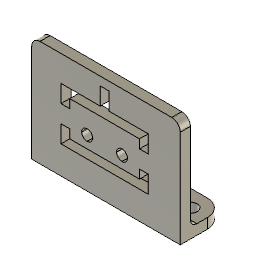
BrandalPilaR v6 (Autodesk Fusion 360 design; units mm, degrees)
Autodesk Fusion 360 part; units mm, degrees
sketch "Sketch1" plane through (0, 0, 0) normal (0, 0, 1) x (1, 0, 0)
  circle A0 centre (0, 0) radius 1.6
  circle A1 centre (0, 0) radius 4
  line L0 (0, 4) -> (20, 4)
  circle A2 centre (20, 0) radius 4
  line L1 (0, -4) -> (20, -4)
  circle A3 centre (20, 0) radius 1.6
  line L2 (-4, 0) -> (-4, -4)
  line L3 (-4, -4) -> (0, -4)
  line L4 (20, -4) -> (24, -4)
  line L5 (24, -4) -> (24, 0)
  dimension "d1" = 3.2
  dimension "d2" = 8
  dimension "d3" = 20
  constraint coincident A0.centre A1.centre
  constraint concentric A0 A1
  constraint coincident A1 L0.start
  constraint horizontal L0
  constraint coincident L0.end A2
  constraint tangent L0 A2
  constraint coincident A1 L1.start
  constraint coincident A2 L1.end
  constraint tangent A2 L1
  constraint horizontal L1
  constraint tangent A1 L1
  constraint tangent A1 L0
  constraint concentric A2 A3
  constraint equal A0 A3
  constraint coincident A1 L2.start
  constraint vertical L2
  constraint horizontal L3
  constraint tangent A1 L2
  constraint tangent A2 L4
  constraint coincident A2 L5.end
  constraint tangent A2 L5
  constraint vertical L5
  measures "d1" diameter of A0
  measures "d2" diameter of A1
  measures "d3" distance of L0.start L0.end
extrude "Extrude1" add sketch "Sketch1" along normal blind 2.4 contours A1 | A1 L0 A2 L1 | A1 L2 L3 | A2 | A2 L4 L5 picked at (-0.2296, -3.1849) picked at (12.0075, 0) picked at (-3.2141, -3.2141) picked at (18.4037, 2.7648) picked at (23.2141, -3.2141)
sketch "Sketch2" plane through (0, -4, 0) normal (0, -1, 0) x (1, 0, 0)
  line L0 (-4, 0) -> (24, 0)
  line L1 (24, 0) -> (24, 2.4)
  line L2 (24, 2.4) -> (-4, 2.4)
  line L3 (-4, 2.4) -> (-4, 0)
  line L4 (-11, 25) -> (24, 25)
  line L5 (24, 25) -> (24, 0)
  line L6 (-4, 0) -> (-11, 0)
  line L7 (-11, 0) -> (-11, 25)
  dimension "d11" = 25
  dimension "d12" = 35
  constraint coincident L0.end L1.start
  constraint perpendicular L0 L5
  constraint coincident L0.start L3.end
  constraint perpendicular L6 L7
  constraint horizontal L4
  constraint vertical L7
  measures "d11" distance of L6.end L4.start
  measures "d12" distance of L4.end L4.start
extrude "Extrude2" add sketch "Sketch2" along normal blind 2.4 contours L0 L1 L2 L3 L5 | L2 L3 L4 L5 L6 L7 picked at (14.6667, 0.8) picked at (3, 17.4667)
fillet "Fillet1" radius 2 2 edges at (24, -5.2, 25) (-11, -5.2, 25)
fillet "Fillet2" radius 1.5 1 edges at (10, -4, 2.4)
sketch "Sketch3" plane through (0, -6.4, 0) normal (0, -1, 0) x (1, 0, 0)
  arc A0 (-9, 25) -> (-11, 23) centre (-9, 23) ccw
  line L0 (-11, 23) -> (-11, 0)
  line L1 (-11, 0) -> (24, 0)
  line L2 (24, 0) -> (24, 23)
  arc A1 (24, 23) -> (22, 25) centre (22, 23) ccw
  line L3 (22, 25) -> (-9, 25)
  spline S0 degree 3 poles (-4.878, 0.7667) (-5.1447, 0.7667) (-5.3826, 0.824) (-5.5918, 0.9388) knots 0 0 0 0 1 1 1 1
  spline S1 degree 3 poles (-5.5918, 0.9388) (-5.801, 1.0535) (-5.9664, 1.2071) (-6.0879, 1.3994) knots 0 0 0 0 1 1 1 1
  spline S2 degree 3 poles (-6.0879, 1.3994) (-6.2094, 1.5952) (-6.2701, 1.8145) (-6.2701, 2.0575) knots 0 0 0 0 1 1 1 1
  spline S3 degree 3 poles (-6.2701, 2.0575) (-6.2701, 2.3005) (-6.2094, 2.5182) (-6.0879, 2.7105) knots 0 0 0 0 1 1 1 1
  spline S4 degree 3 poles (-6.0879, 2.7105) (-5.9664, 2.9062) (-5.801, 3.0615) (-5.5918, 3.1762) knots 0 0 0 0 1 1 1 1
  spline S5 degree 3 poles (-5.5918, 3.1762) (-5.3826, 3.291) (-5.1447, 3.3483) (-4.878, 3.3483) knots 0 0 0 0 1 1 1 1
  line L4 (-4.878, 3.3483) -> (-4.5642, 3.3483)
  line L5 (-4.5642, 3.3483) -> (-4.5642, 2.8523)
  line L6 (-4.5642, 2.8523) -> (-4.8882, 2.8523)
  spline S6 degree 3 poles (-4.8882, 2.8523) (-5.0434, 2.8523) (-5.1818, 2.8168) (-5.3033, 2.746) knots 0 0 0 0 1 1 1 1
  spline S7 degree 3 poles (-5.3033, 2.746) (-5.4214, 2.6784) (-5.5142, 2.584) (-5.5817, 2.4625) knots 0 0 0 0 1 1 1 1
  spline S8 degree 3 poles (-5.5817, 2.4625) (-5.6492, 2.341) (-5.6829, 2.206) (-5.6829, 2.0575) knots 0 0 0 0 1 1 1 1
  spline S9 degree 3 poles (-5.6829, 2.0575) (-5.6829, 1.909) (-5.6492, 1.774) (-5.5817, 1.6526) knots 0 0 0 0 1 1 1 1
  spline S10 degree 3 poles (-5.5817, 1.6526) (-5.5142, 1.5311) (-5.4214, 1.4349) (-5.3033, 1.364) knots 0 0 0 0 1 1 1 1
  spline S11 degree 3 poles (-5.3033, 1.364) (-5.1818, 1.2965) (-5.0434, 1.2628) (-4.8882, 1.2628) knots 0 0 0 0 1 1 1 1
  line L7 (-4.8882, 1.2628) -> (-4.5642, 1.2628)
  line L8 (-4.5642, 1.2628) -> (-4.5642, 0.7667)
  line L9 (-4.5642, 0.7667) -> (-4.878, 0.7667)
  line L10 (-4.057, 0.7667) -> (-4.057, 4.462)
  line L11 (-4.057, 4.462) -> (-3.4748, 4.462)
  line L12 (-3.4748, 4.462) -> (-3.4748, 3.0902)
  spline S12 degree 3 poles (-3.4748, 3.0902) (-3.3702, 3.2015) (-3.2487, 3.2825) (-3.1104, 3.3332) knots 0 0 0 0 1 1 1 1
  spline S13 degree 3 poles (-3.1104, 3.3332) (-2.972, 3.3838) (-2.8319, 3.4091) (-2.6902, 3.4091) knots 0 0 0 0 1 1 1 1
  spline S14 degree 3 poles (-2.6902, 3.4091) (-2.454, 3.4091) (-2.2532, 3.3585) (-2.0878, 3.2572) knots 0 0 0 0 1 1 1 1
  spline S15 degree 3 poles (-2.0878, 3.2572) (-1.9191, 3.1593) (-1.7909, 3.0227) (-1.7031, 2.8472) knots 0 0 0 0 1 1 1 1
  spline S16 degree 3 poles (-1.7031, 2.8472) (-1.6154, 2.6751) (-1.5715, 2.4777) (-1.5715, 2.2549) knots 0 0 0 0 1 1 1 1
  line L13 (-1.5715, 2.2549) -> (-1.5715, 0.7667)
  line L14 (-1.5715, 0.7667) -> (-2.1486, 0.7667)
  line L15 (-2.1486, 0.7667) -> (-2.1486, 2.2499)
  spline S17 degree 3 poles (-2.1486, 2.2499) (-2.1486, 2.3815) (-2.1806, 2.4962) (-2.2447, 2.5941) knots 0 0 0 0 1 1 1 1
  spline S18 degree 3 poles (-2.2447, 2.5941) (-2.3055, 2.6953) (-2.3865, 2.7729) (-2.4877, 2.8269) knots 0 0 0 0 1 1 1 1
  spline S19 degree 3 poles (-2.4877, 2.8269) (-2.5856, 2.8843) (-2.6953, 2.913) (-2.8168, 2.913) knots 0 0 0 0 1 1 1 1
  spline S20 degree 3 poles (-2.8168, 2.913) (-2.9315, 2.913) (-3.0395, 2.886) (-3.1407, 2.832) knots 0 0 0 0 1 1 1 1
  spline S21 degree 3 poles (-3.1407, 2.832) (-3.242, 2.778) (-3.323, 2.7021) (-3.3837, 2.6042) knots 0 0 0 0 1 1 1 1
  spline S22 degree 3 poles (-3.3837, 2.6042) (-3.4445, 2.5063) (-3.4748, 2.395) (-3.4748, 2.2701) knots 0 0 0 0 1 1 1 1
  line L16 (-3.4748, 2.2701) -> (-3.4748, 0.7667)
  line L17 (-3.4748, 0.7667) -> (-4.057, 0.7667)
  spline S23 degree 3 poles (0.1744, 0.7059) (-0.0719, 0.7059) (-0.2845, 0.7667) (-0.4634, 0.8882) knots 0 0 0 0 1 1 1 1
  spline S24 degree 3 poles (-0.4634, 0.8882) (-0.6423, 1.0097) (-0.7806, 1.1717) (-0.8785, 1.3741) knots 0 0 0 0 1 1 1 1
  spline S25 degree 3 poles (-0.8785, 1.3741) (-0.9729, 1.58) (-1.0202, 1.8061) (-1.0202, 2.0525) knots 0 0 0 0 1 1 1 1
  spline S26 degree 3 poles (-1.0202, 2.0525) (-1.0202, 2.3089) (-0.9662, 2.5384) (-0.8582, 2.7409) knots 0 0 0 0 1 1 1 1
  spline S27 degree 3 poles (-0.8582, 2.7409) (-0.7469, 2.9467) (-0.5899, 3.1087) (-0.3874, 3.2269) knots 0 0 0 0 1 1 1 1
  spline S28 degree 3 poles (-0.3874, 3.2269) (-0.1816, 3.3483) (0.0631, 3.4091) (0.3466, 3.4091) knots 0 0 0 0 1 1 1 1
  spline S29 degree 3 poles (0.3466, 3.4091) (0.6267, 3.4091) (0.8646, 3.3483) (1.0603, 3.2269) knots 0 0 0 0 1 1 1 1
  spline S30 degree 3 poles (1.0603, 3.2269) (1.2594, 3.1087) (1.4113, 2.9467) (1.5159, 2.7409) knots 0 0 0 0 1 1 1 1
  spline S31 degree 3 poles (1.5159, 2.7409) (1.6239, 2.5384) (1.6779, 2.3123) (1.6779, 2.0626) knots 0 0 0 0 1 1 1 1
  line L18 (1.6779, 2.0626) -> (1.6779, 0.7667)
  line L19 (1.6779, 0.7667) -> (1.0957, 0.7667)
  line L20 (1.0957, 0.7667) -> (1.0957, 1.2476)
  line L21 (1.0957, 1.2476) -> (1.0856, 1.2476)
  spline S32 degree 3 poles (1.0856, 1.2476) (1.035, 1.1531) (0.9692, 1.0637) (0.8882, 0.9793) knots 0 0 0 0 1 1 1 1
  spline S33 degree 3 poles (0.8882, 0.9793) (0.8072, 0.8983) (0.7077, 0.8325) (0.5895, 0.7819) knots 0 0 0 0 1 1 1 1
  spline S34 degree 3 poles (0.5895, 0.7819) (0.4714, 0.7313) (0.3331, 0.7059) (0.1744, 0.7059) knots 0 0 0 0 1 1 1 1
  spline S35 degree 3 poles (0.3314, 1.202) (0.4832, 1.202) (0.6148, 1.2391) (0.7262, 1.3134) knots 0 0 0 0 1 1 1 1
  spline S36 degree 3 poles (0.7262, 1.3134) (0.8409, 1.391) (0.9287, 1.4939) (0.9894, 1.6222) knots 0 0 0 0 1 1 1 1
  spline S37 degree 3 poles (0.9894, 1.6222) (1.0535, 1.7538) (1.0856, 1.9006) (1.0856, 2.0626) knots 0 0 0 0 1 1 1 1
  spline S38 degree 3 poles (1.0856, 2.0626) (1.0856, 2.2246) (1.0552, 2.368) (0.9945, 2.4929) knots 0 0 0 0 1 1 1 1
  spline S39 degree 3 poles (0.9945, 2.4929) (0.9338, 2.6211) (0.8477, 2.7223) (0.7363, 2.7966) knots 0 0 0 0 1 1 1 1
  spline S40 degree 3 poles (0.7363, 2.7966) (0.625, 2.8742) (0.4917, 2.913) (0.3364, 2.913) knots 0 0 0 0 1 1 1 1
  spline S41 degree 3 poles (0.3364, 2.913) (0.1744, 2.913) (0.0361, 2.8742) (-0.0787, 2.7966) knots 0 0 0 0 1 1 1 1
  spline S42 degree 3 poles (-0.0787, 2.7966) (-0.1934, 2.7223) (-0.2811, 2.6211) (-0.3419, 2.4929) knots 0 0 0 0 1 1 1 1
  spline S43 degree 3 poles (-0.3419, 2.4929) (-0.4026, 2.3646) (-0.433, 2.2195) (-0.433, 2.0575) knots 0 0 0 0 1 1 1 1
  spline S44 degree 3 poles (-0.433, 2.0575) (-0.433, 1.8989) (-0.4026, 1.7538) (-0.3419, 1.6222) knots 0 0 0 0 1 1 1 1
  spline S45 degree 3 poles (-0.3419, 1.6222) (-0.2811, 1.4939) (-0.1951, 1.391) (-0.0837, 1.3134) knots 0 0 0 0 1 1 1 1
  spline S46 degree 3 poles (-0.0837, 1.3134) (0.031, 1.2391) (0.1694, 1.202) (0.3314, 1.202) knots 0 0 0 0 1 1 1 1
  line L22 (2.3947, 0.7667) -> (2.3947, 4.3101)
  line L23 (2.3947, 4.3101) -> (4.3486, 4.3101)
  spline S47 degree 3 poles (4.3486, 4.3101) (4.5241, 4.3101) (4.6794, 4.2713) (4.8143, 4.1937) knots 0 0 0 0 1 1 1 1
  spline S48 degree 3 poles (4.8143, 4.1937) (4.9527, 4.1161) (5.0607, 4.0098) (5.1383, 3.8748) knots 0 0 0 0 1 1 1 1
  spline S49 degree 3 poles (5.1383, 3.8748) (5.2193, 3.7398) (5.2598, 3.5829) (5.2598, 3.404) knots 0 0 0 0 1 1 1 1
  spline S50 degree 3 poles (5.2598, 3.404) (5.2598, 3.2859) (5.2345, 3.1728) (5.1839, 3.0649) knots 0 0 0 0 1 1 1 1
  spline S51 degree 3 poles (5.1839, 3.0649) (5.1366, 2.9569) (5.0708, 2.8624) (4.9864, 2.7814) knots 0 0 0 0 1 1 1 1
  spline S52 degree 3 poles (4.9864, 2.7814) (4.9021, 2.7038) (4.8042, 2.643) (4.6928, 2.5992) knots 0 0 0 0 1 1 1 1
  spline S53 degree 3 poles (4.6928, 2.5992) (4.8211, 2.562) (4.9341, 2.4996) (5.032, 2.4119) knots 0 0 0 0 1 1 1 1
  spline S54 degree 3 poles (5.032, 2.4119) (5.1332, 2.3241) (5.2125, 2.2195) (5.2699, 2.098) knots 0 0 0 0 1 1 1 1
  spline S55 degree 3 poles (5.2699, 2.098) (5.3273, 1.9765) (5.356, 1.8466) (5.356, 1.7082) knots 0 0 0 0 1 1 1 1
  spline S56 degree 3 poles (5.356, 1.7082) (5.356, 1.526) (5.3138, 1.364) (5.2294, 1.2223) knots 0 0 0 0 1 1 1 1
  spline S57 degree 3 poles (5.2294, 1.2223) (5.1484, 1.0805) (5.0354, 0.9692) (4.8903, 0.8882) knots 0 0 0 0 1 1 1 1
  spline S58 degree 3 poles (4.8903, 0.8882) (4.7485, 0.8072) (4.5848, 0.7667) (4.3992, 0.7667) knots 0 0 0 0 1 1 1 1
  line L24 (4.3992, 0.7667) -> (2.3947, 0.7667)
  line L25 (2.9971, 1.3033) -> (4.2373, 1.3033)
  spline S59 degree 3 poles (4.2373, 1.3033) (4.3385, 1.3033) (4.4279, 1.3252) (4.5055, 1.3691) knots 0 0 0 0 1 1 1 1
  spline S60 degree 3 poles (4.5055, 1.3691) (4.5832, 1.4163) (4.6422, 1.4787) (4.6827, 1.5564) knots 0 0 0 0 1 1 1 1
  spline S61 degree 3 poles (4.6827, 1.5564) (4.7266, 1.6374) (4.7485, 1.7217) (4.7485, 1.8095) knots 0 0 0 0 1 1 1 1
  spline S62 degree 3 poles (4.7485, 1.8095) (4.7485, 1.9006) (4.7266, 1.9832) (4.6827, 2.0575) knots 0 0 0 0 1 1 1 1
  spline S63 degree 3 poles (4.6827, 2.0575) (4.6389, 2.1351) (4.5781, 2.1976) (4.5005, 2.2448) knots 0 0 0 0 1 1 1 1
  spline S64 degree 3 poles (4.5005, 2.2448) (4.4229, 2.292) (4.3317, 2.3157) (4.2271, 2.3157) knots 0 0 0 0 1 1 1 1
  line L26 (4.2271, 2.3157) -> (2.9971, 2.3157)
  line L27 (2.9971, 2.3157) -> (2.9971, 1.3033)
  line L28 (2.9971, 2.8269) -> (4.1613, 2.8269)
  spline S65 degree 3 poles (4.1613, 2.8269) (4.2558, 2.8269) (4.3402, 2.8489) (4.4144, 2.8928) knots 0 0 0 0 1 1 1 1
  spline S66 degree 3 poles (4.4144, 2.8928) (4.4921, 2.9366) (4.5511, 2.994) (4.5916, 3.0649) knots 0 0 0 0 1 1 1 1
  spline S67 degree 3 poles (4.5916, 3.0649) (4.6355, 3.1391) (4.6574, 3.2184) (4.6574, 3.3028) knots 0 0 0 0 1 1 1 1
  spline S68 degree 3 poles (4.6574, 3.3028) (4.6574, 3.3905) (4.6372, 3.4698) (4.5967, 3.5407) knots 0 0 0 0 1 1 1 1
  spline S69 degree 3 poles (4.5967, 3.5407) (4.5562, 3.6116) (4.4988, 3.6689) (4.4246, 3.7128) knots 0 0 0 0 1 1 1 1
  spline S70 degree 3 poles (4.4246, 3.7128) (4.3537, 3.7567) (4.271, 3.7786) (4.1765, 3.7786) knots 0 0 0 0 1 1 1 1
  line L29 (4.1765, 3.7786) -> (2.9971, 3.7786)
  line L30 (2.9971, 3.7786) -> (2.9971, 2.8269)
  spline S71 degree 3 poles (7.144, 0.7059) (6.8774, 0.7059) (6.6411, 0.765) (6.4353, 0.8831) knots 0 0 0 0 1 1 1 1
  spline S72 degree 3 poles (6.4353, 0.8831) (6.2295, 1.0046) (6.0658, 1.1666) (5.9443, 1.3691) knots 0 0 0 0 1 1 1 1
  spline S73 degree 3 poles (5.9443, 1.3691) (5.8262, 1.5749) (5.7671, 1.8044) (5.7671, 2.0575) knots 0 0 0 0 1 1 1 1
  spline S74 degree 3 poles (5.7671, 2.0575) (5.7671, 2.3106) (5.8262, 2.5384) (5.9443, 2.7409) knots 0 0 0 0 1 1 1 1
  spline S75 degree 3 poles (5.9443, 2.7409) (6.0658, 2.9467) (6.2295, 3.1087) (6.4353, 3.2269) knots 0 0 0 0 1 1 1 1
  spline S76 degree 3 poles (6.4353, 3.2269) (6.6411, 3.3483) (6.8774, 3.4091) (7.144, 3.4091) knots 0 0 0 0 1 1 1 1
  spline S77 degree 3 poles (7.144, 3.4091) (7.4072, 3.4091) (7.6418, 3.3483) (7.8476, 3.2269) knots 0 0 0 0 1 1 1 1
  spline S78 degree 3 poles (7.8476, 3.2269) (8.0535, 3.1087) (8.2154, 2.9484) (8.3336, 2.746) knots 0 0 0 0 1 1 1 1
  spline S79 degree 3 poles (8.3336, 2.746) (8.4551, 2.5435) (8.5158, 2.314) (8.5158, 2.0575) knots 0 0 0 0 1 1 1 1
  spline S80 degree 3 poles (8.5158, 2.0575) (8.5158, 1.8044) (8.4551, 1.5749) (8.3336, 1.3691) knots 0 0 0 0 1 1 1 1
  spline S81 degree 3 poles (8.3336, 1.3691) (8.2154, 1.1666) (8.0535, 1.0046) (7.8476, 0.8831) knots 0 0 0 0 1 1 1 1
  spline S82 degree 3 poles (7.8476, 0.8831) (7.6418, 0.765) (7.4072, 0.7059) (7.144, 0.7059) knots 0 0 0 0 1 1 1 1
  spline S83 degree 3 poles (7.144, 1.202) (7.3026, 1.202) (7.4409, 1.2391) (7.5591, 1.3134) knots 0 0 0 0 1 1 1 1
  spline S84 degree 3 poles (7.5591, 1.3134) (7.6772, 1.391) (7.7683, 1.4939) (7.8324, 1.6222) knots 0 0 0 0 1 1 1 1
  spline S85 degree 3 poles (7.8324, 1.6222) (7.8965, 1.7504) (7.9286, 1.8955) (7.9286, 2.0575) knots 0 0 0 0 1 1 1 1
  spline S86 degree 3 poles (7.9286, 2.0575) (7.9286, 2.2161) (7.8965, 2.3595) (7.8324, 2.4878) knots 0 0 0 0 1 1 1 1
  spline S87 degree 3 poles (7.8324, 2.4878) (7.7683, 2.6194) (7.6772, 2.7223) (7.5591, 2.7966) knots 0 0 0 0 1 1 1 1
  spline S88 degree 3 poles (7.5591, 2.7966) (7.4409, 2.8742) (7.3026, 2.913) (7.144, 2.913) knots 0 0 0 0 1 1 1 1
  spline S89 degree 3 poles (7.144, 2.913) (6.982, 2.913) (6.842, 2.8742) (6.7238, 2.7966) knots 0 0 0 0 1 1 1 1
  spline S90 degree 3 poles (6.7238, 2.7966) (6.6091, 2.7223) (6.518, 2.6211) (6.4505, 2.4929) knots 0 0 0 0 1 1 1 1
  spline S91 degree 3 poles (6.4505, 2.4929) (6.3864, 2.3646) (6.3543, 2.2195) (6.3543, 2.0575) knots 0 0 0 0 1 1 1 1
  spline S92 degree 3 poles (6.3543, 2.0575) (6.3543, 1.8989) (6.3864, 1.7538) (6.4505, 1.6222) knots 0 0 0 0 1 1 1 1
  spline S93 degree 3 poles (6.4505, 1.6222) (6.518, 1.4939) (6.6091, 1.391) (6.7238, 1.3134) knots 0 0 0 0 1 1 1 1
  spline S94 degree 3 poles (6.7238, 1.3134) (6.842, 1.2391) (6.982, 1.202) (7.144, 1.202) knots 0 0 0 0 1 1 1 1
  spline S95 degree 3 poles (9.8599, 0.7667) (9.6304, 0.7667) (9.4498, 0.8325) (9.3182, 0.9641) knots 0 0 0 0 1 1 1 1
  spline S96 degree 3 poles (9.3182, 0.9641) (9.19, 1.0957) (9.1259, 1.2746) (9.1259, 1.5007) knots 0 0 0 0 1 1 1 1
  line L31 (9.1259, 1.5007) -> (9.1259, 3.9963)
  line L32 (9.1259, 3.9963) -> (9.7029, 3.9963)
  line L33 (9.7029, 3.9963) -> (9.7029, 1.526)
  spline S97 degree 3 poles (9.7029, 1.526) (9.7029, 1.4484) (9.7265, 1.3843) (9.7738, 1.3336) knots 0 0 0 0 1 1 1 1
  spline S98 degree 3 poles (9.7738, 1.3336) (9.8211, 1.2864) (9.8835, 1.2628) (9.9611, 1.2628) knots 0 0 0 0 1 1 1 1
  line L34 (9.9611, 1.2628) -> (10.5027, 1.2628)
  line L35 (10.5027, 1.2628) -> (10.5027, 0.7667)
  line L36 (10.5027, 0.7667) -> (9.8599, 0.7667)
  line L37 (8.6804, 2.8523) -> (8.6804, 3.3483)
  line L38 (8.6804, 3.3483) -> (10.5078, 3.3483)
  line L39 (10.5078, 3.3483) -> (10.5078, 2.8523)
  line L40 (10.5078, 2.8523) -> (8.6804, 2.8523)
  line L41 (11.0449, 0.7667) -> (11.0449, 1.2628)
  line L42 (11.0449, 1.2628) -> (12.2902, 1.2628)
  spline S99 degree 3 poles (12.2902, 1.2628) (12.3509, 1.2628) (12.4033, 1.2763) (12.4471, 1.3033) knots 0 0 0 0 1 1 1 1
  spline S100 degree 3 poles (12.4471, 1.3033) (12.4944, 1.3302) (12.5298, 1.3657) (12.5534, 1.4096) knots 0 0 0 0 1 1 1 1
  spline S101 degree 3 poles (12.5534, 1.4096) (12.5804, 1.4534) (12.5939, 1.499) (12.5939, 1.5462) knots 0 0 0 0 1 1 1 1
  spline S102 degree 3 poles (12.5939, 1.5462) (12.5939, 1.6002) (12.5821, 1.6475) (12.5585, 1.688) knots 0 0 0 0 1 1 1 1
  spline S103 degree 3 poles (12.5585, 1.688) (12.5349, 1.7285) (12.5011, 1.7605) (12.4572, 1.7842) knots 0 0 0 0 1 1 1 1
  spline S104 degree 3 poles (12.4572, 1.7842) (12.4134, 1.8111) (12.3628, 1.8247) (12.3054, 1.8247) knots 0 0 0 0 1 1 1 1
  line L43 (12.3054, 1.8247) -> (11.7992, 1.8247)
  spline S105 degree 3 poles (11.7992, 1.8247) (11.6338, 1.8247) (11.487, 1.8516) (11.3588, 1.9057) knots 0 0 0 0 1 1 1 1
  spline S106 degree 3 poles (11.3588, 1.9057) (11.2305, 1.9596) (11.1293, 2.0423) (11.0551, 2.1537) knots 0 0 0 0 1 1 1 1
  spline S107 degree 3 poles (11.0551, 2.1537) (10.9808, 2.2684) (10.9437, 2.4119) (10.9437, 2.584) knots 0 0 0 0 1 1 1 1
  spline S108 degree 3 poles (10.9437, 2.584) (10.9437, 2.7223) (10.9774, 2.8489) (11.0449, 2.9636) knots 0 0 0 0 1 1 1 1
  spline S109 degree 3 poles (11.0449, 2.9636) (11.1158, 3.0784) (11.2103, 3.1712) (11.3284, 3.242) knots 0 0 0 0 1 1 1 1
  spline S110 degree 3 poles (11.3284, 3.242) (11.4465, 3.3129) (11.5798, 3.3483) (11.7283, 3.3483) knots 0 0 0 0 1 1 1 1
  line L44 (11.7283, 3.3483) -> (12.928, 3.3483)
  line L45 (12.928, 3.3483) -> (12.928, 2.8523)
  line L46 (12.928, 2.8523) -> (11.784, 2.8523)
  spline S111 degree 3 poles (11.784, 2.8523) (11.7064, 2.8523) (11.6423, 2.8269) (11.5916, 2.7763) knots 0 0 0 0 1 1 1 1
  spline S112 degree 3 poles (11.5916, 2.7763) (11.541, 2.7291) (11.5157, 2.67) (11.5157, 2.5992) knots 0 0 0 0 1 1 1 1
  spline S113 degree 3 poles (11.5157, 2.5992) (11.5157, 2.5316) (11.541, 2.4726) (11.5916, 2.422) knots 0 0 0 0 1 1 1 1
  spline S114 degree 3 poles (11.5916, 2.422) (11.6423, 2.3714) (11.7098, 2.3461) (11.7941, 2.3461) knots 0 0 0 0 1 1 1 1
  line L47 (11.7941, 2.3461) -> (12.2851, 2.3461)
  spline S115 degree 3 poles (12.2851, 2.3461) (12.4707, 2.3461) (12.6294, 2.3173) (12.761, 2.26) knots 0 0 0 0 1 1 1 1
  spline S116 degree 3 poles (12.761, 2.26) (12.8926, 2.2026) (12.9921, 2.1166) (13.0596, 2.0018) knots 0 0 0 0 1 1 1 1
  spline S117 degree 3 poles (13.0596, 2.0018) (13.1305, 1.8871) (13.1659, 1.742) (13.1659, 1.5665) knots 0 0 0 0 1 1 1 1
  spline S118 degree 3 poles (13.1659, 1.5665) (13.1659, 1.4248) (13.1305, 1.2914) (13.0596, 1.1666) knots 0 0 0 0 1 1 1 1
  spline S119 degree 3 poles (13.0596, 1.1666) (12.9888, 1.0451) (12.8909, 0.9472) (12.766, 0.873) knots 0 0 0 0 1 1 1 1
  spline S120 degree 3 poles (12.766, 0.873) (12.6445, 0.8021) (12.5062, 0.7667) (12.3509, 0.7667) knots 0 0 0 0 1 1 1 1
  line L48 (12.3509, 0.7667) -> (11.0449, 0.7667)
  line L49 (16.8144, 3.9303) -> (17.505, 3.9304)
  line L50 (17.505, 3.9304) -> (19.5378, 0.6823)
  line L51 (19.5378, 0.6823) -> (18.8469, 0.6824)
  line L52 (18.8469, 0.6824) -> (16.8144, 3.9303)
  line L53 (16.8144, 0.6822) -> (17.505, 0.6821)
  line L54 (17.505, 0.6821) -> (19.5378, 3.9302)
  line L55 (19.5378, 3.9302) -> (18.8469, 3.9301)
  line L56 (18.8469, 3.9301) -> (16.8144, 0.6822)
  line L57 (13.7319, 3.917) -> (14.3251, 3.917)
  line L58 (14.3251, 3.917) -> (14.3251, 0.6807)
  line L59 (14.3251, 0.6807) -> (13.7319, 0.6807)
  line L60 (13.7319, 0.6807) -> (13.7319, 3.917)
  line L61 (13.8114, 3.6203) -> (14.3251, 3.917)
  line L62 (14.3251, 3.917) -> (15.0964, 2.5783)
  line L63 (15.0964, 2.5783) -> (15.0964, 1.5303)
  line L64 (15.0964, 1.5303) -> (14.5828, 2.2848)
  line L65 (14.5828, 2.2848) -> (13.8114, 3.6203)
  line L66 (16.375, 3.6203) -> (15.8613, 3.917)
  line L67 (15.8613, 3.917) -> (15.0964, 2.5783)
  line L68 (15.0964, 2.5783) -> (15.0964, 1.5303)
  line L69 (15.0964, 1.5303) -> (15.6039, 2.2848)
  line L70 (15.6039, 2.2848) -> (16.375, 3.6203)
  line L71 (16.4545, 3.917) -> (15.8613, 3.917)
  line L72 (15.8613, 3.917) -> (15.8613, 0.6807)
  line L73 (15.8613, 0.6807) -> (16.4545, 0.6807)
  line L74 (16.4545, 0.6807) -> (16.4545, 3.917)
  line L75 (7.2182, 23.0002) -> (5.1656, 23.0002)
  line L76 (5.1656, 23.0002) -> (5.1656, 18.8953)
  line L77 (5.1656, 18.8953) -> (7.2182, 18.8953)
  line L78 (7.2182, 18.8953) -> (7.2182, 23.0002)
  line L79 (16.4545, 16.8424) -> (16.4545, 18.895)
  line L80 (16.4545, 18.895) -> (-4.0699, 18.895)
  line L81 (-4.0699, 18.895) -> (-4.0699, 16.8424)
  line L82 (-4.0699, 16.8424) -> (16.4545, 16.8424)
  line L83 (16.4545, 6.5801) -> (16.4545, 8.6328)
  line L84 (16.4545, 8.6328) -> (-4.0699, 8.6328)
  line L85 (-4.0699, 8.6328) -> (-4.0699, 6.5801)
  line L86 (-4.0699, 6.5801) -> (16.4545, 6.5801)
  spline S121 degree 3 poles (2.0864, 10.1722) (2.7943, 10.1722) (3.3682, 10.7461) (3.3682, 11.4541) knots 0 0 0 0 1 1 1 1
  spline S122 degree 3 poles (3.3682, 11.4541) (3.3682, 12.1621) (2.7943, 12.736) (2.0864, 12.736) knots 0 0 0 0 1 1 1 1
  spline S123 degree 3 poles (2.0864, 12.736) (1.3784, 12.736) (0.8045, 12.1621) (0.8045, 11.4541) knots 0 0 0 0 1 1 1 1
  spline S124 degree 3 poles (0.8045, 11.4541) (0.8045, 10.7461) (1.3784, 10.1722) (2.0864, 10.1722) knots 0 0 0 0 1 1 1 1
  line L87 (-2.0179, 18.8952) -> (-4.0699, 18.895)
  line L88 (-4.0699, 18.895) -> (-4.0706, 14.7903)
  line L89 (-4.0706, 14.7903) -> (-2.0179, 14.7903)
  line L90 (-2.0179, 14.7903) -> (-2.0179, 18.8952)
  line L91 (16.4545, 18.895) -> (14.4013, 18.8952)
  line L92 (14.4013, 18.8952) -> (14.4013, 14.7903)
  line L93 (14.4013, 14.7903) -> (16.4539, 14.7903)
  line L94 (16.4539, 14.7903) -> (16.4545, 18.895)
  line L95 (-2.0179, 10.6855) -> (-4.0706, 10.6855)
  line L96 (-4.0706, 10.6855) -> (-4.0699, 6.5801)
  line L97 (-4.0699, 6.5801) -> (-2.0179, 6.5806)
  line L98 (-2.0179, 6.5806) -> (-2.0179, 10.6855)
  line L99 (16.4539, 10.6855) -> (14.4013, 10.6855)
  line L100 (14.4013, 10.6855) -> (14.4013, 6.5806)
  line L101 (14.4013, 6.5806) -> (16.4545, 6.5801)
  line L102 (16.4545, 6.5801) -> (16.4539, 10.6855)
  spline S125 degree 3 poles (10.2964, 10.1736) (11.0044, 10.1736) (11.5783, 10.7475) (11.5783, 11.4555) knots 0 0 0 0 1 1 1 1
  spline S126 degree 3 poles (11.5783, 11.4555) (11.5783, 12.1634) (11.0044, 12.7374) (10.2964, 12.7374) knots 0 0 0 0 1 1 1 1
  spline S127 degree 3 poles (10.2964, 12.7374) (9.5884, 12.7374) (9.0145, 12.1634) (9.0145, 11.4555) knots 0 0 0 0 1 1 1 1
  spline S128 degree 3 poles (9.0145, 11.4555) (9.0145, 10.7475) (9.5884, 10.1736) (10.2964, 10.1736) knots 0 0 0 0 1 1 1 1
extrude "Extrude3" cut sketch "Sketch3" against normal up to surface (2.4 mm away) contours L75 L76 L77 L78 | L80 L82 L92 L94 | L82 L92 L93 L94 | L80 L82 L90 L92 | L80 L81 L82 L90 | L81 L82 L88 L89 L90 | L84 L86 L97 L98 L100 L101 | L84 L100 L101 L102 | L84 L85 L95 L96 L98 | L84 L85 L97 L98 | L84 L99 L100 L102 | S121 S122 S123 S124 | S125 S126 S127 S128 picked at (5.8498, 21.6319) picked at (15.77, 18.2108) picked at (15.7698, 16.1584) picked at (3.4551, 18.2108) picked at (-2.7019, 17.5266) picked at (-3.3861, 15.4743) picked at (3.4551, 7.2646) picked at (15.77, 7.2645) picked at (-3.3861, 10.0013) picked at (-3.3859, 7.2645) picked at (15.7698, 9.317) picked at (1.7879, 11.1483) picked at (10.5949, 11.7613)
extrude "Extrude4" cut 1 faces at (5.8498, -5.6, 18.8953) along direction (0, 0, -1) blind 1
